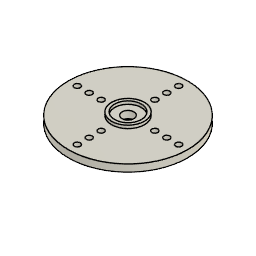
Savöx_SH_0255 MG_micro_servo_horn (Autodesk Fusion 360 design; units mm, degrees)
description: Spur Gear; Module: 0.217; Num Teeth: 21; Pressure Angle: 20.0; Backlash: 0.00 mm
part number: 2026-07-12-11-53-48-100
Autodesk Fusion 360 part; units mm, degrees
sketch "Horn body" plane through (0, 0, 0) normal (0, 0, 1) x (1, 0, 0)
  circle A0 centre (0, 0) radius 10
  dimension "d1" = 20
  constraint coincident A0.centre origin
  measures "d1" diameter of A0
extrude "Extrude1" add sketch "Horn body" along normal blind 1.2 makes body 1
sketch "Connector" plane through (0, 0, 0) normal (0, 0, -1) x (1, 0, 0)
  circle A0 centre (0, 0) radius 10
  circle A1 centre (0, 0) radius 3.5
  dimension "d5" = 7
  constraint coincident A0.centre A1.centre
  measures "d5" diameter of A1
extrude "Extrude2" add sketch "Connector" along normal blind 3 contours A1 bodies 1
sketch "Screw hole" plane through (0, 0, 1.2) normal (0, 0, 1) x (-1, 0, 0)
  circle A0 centre (0, 0) radius 10
  circle A1 centre (0, 0) radius 2.75
  circle A2 centre (0, 0) radius 2.25
  circle A3 centre (0, 0) radius 1
  dimension "d8" = 5.5
  dimension "d9" = 4.5
  dimension "d10" = 2
  constraint coincident A0.centre A1.centre
  constraint concentric A2 A3
  measures "d8" diameter of A1
  measures "d9" diameter of A2
  measures "d10" diameter of A3
extrude "Extrude3" add sketch "Screw hole" along normal blind 0.5 contours A1 bodies 1
extrude "Extrude4" cut sketch "Screw hole" against normal blind 1.2 contours A3 bodies 1
sketch "Top small holes" plane through (0, 0, 1.2) normal (0, 0, 1) x (-1, 0, 0)
  circle A0 centre (0, 0) radius 10
  circle A1 centre (0, 0) radius 2.75
  circle A2 centre (0, -8.5) radius 0.5
  circle A3 centre (0, -6.5) radius 0.5
  circle A4 centre (0, -4.5) radius 0.5
  dimension "d15" = 1
  dimension "d16" = 1
  dimension "d17" = 1
  dimension "d19" = 8.5
  dimension "d20" = 6.5
  dimension "d21" = 4.5
  measures "d15" diameter of A2
  measures "d16" diameter of A3
  measures "d17" diameter of A4
  measures "d19" distance of A0.centre A2.centre
  measures "d20" distance of A0.centre A3.centre
  measures "d21" distance of A0.centre A4.centre
extrude "Extrude5" cut sketch "Top small holes" against normal blind 1.2 contours A2 | A3 | A4 bodies 1
pattern_circular "C-Pattern1" count 4 over 360 about axis through (0, 0, 1.75) along (0, 0, 1) of "Extrude5"
sketch "Base Circle" plane through (0, 0, 0) normal (0, 0, 1) x (1, 0, 0) in component "Savöx SH 0255 MG Micro Servo Gear"
  circle A0 centre (0, 0) radius 2.0274
extrude "Extrude1'" add sketch "Base Circle" along normal blind 3 separate body makes body 2 in component "Savöx SH 0255 MG Micro Servo Gear"
sketch "Gear Tooth" plane through (0, 0, 0) normal (0, 0, 1) x (1, 0, 0) in component "Savöx SH 0255 MG Micro Servo Gear"
  spline S0 degree 5 poles (2.1325, -0.1918) (2.1335, -0.1919) (2.1355, -0.1921) (2.1386, -0.1922) (2.1427, -0.1923) (2.1478, -0.1921) (2.1529, -0.1919) (2.1581, -0.1915) (2.1632, -0.191) (2.1683, -0.1906) (2.1735, -0.1901) (2.1787, -0.1895) (2.1838, -0.1889) (2.189, -0.1882) (2.1941, -0.1875) (2.1993, -0.1867) (2.2045, -0.1858) (2.2097, -0.1849) (2.2148, -0.1839) (2.22, -0.1829) (2.2252, -0.1818) (2.2304, -0.1807) (2.2356, -0.1796) (2.2407, -0.1784) (2.2459, -0.1772) (2.2511, -0.1759) (2.2563, -0.1746) (2.2615, -0.1732) (2.2667, -0.1718) (2.2719, -0.1703) (2.2771, -0.1689) (2.2823, -0.1674) (2.2875, -0.1658) (2.2927, -0.1642) (2.2979, -0.1626) (2.3031, -0.1609) (2.3083, -0.1592) (2.3134, -0.1575) (2.3186, -0.1557) (2.3238, -0.1539) (2.329, -0.152) (2.3342, -0.1502) (2.3394, -0.1482) (2.3446, -0.1463) (2.3498, -0.1443) (2.355, -0.1423) (2.3602, -0.1403) (2.3654, -0.1382) (2.3705, -0.1361) (2.3757, -0.1339) (2.3809, -0.1317) (2.3861, -0.1295) (2.3913, -0.1273) (2.3964, -0.125) (2.4016, -0.1227) (2.4068, -0.1204) (2.412, -0.118) (2.4171, -0.1156) (2.4223, -0.1132) (2.4275, -0.1107) (2.4326, -0.1082) (2.4378, -0.1057) (2.4429, -0.1032) (2.4481, -0.1006) (2.4532, -0.098) (2.4584, -0.0953) (2.4635, -0.0927) (2.4687, -0.09) (2.4738, -0.0872) (2.479, -0.0845) (2.4841, -0.0817) (2.4882, -0.0794) (2.4913, -0.0777) (2.4933, -0.0766) (2.4943, -0.076) knots 0 0 0 0 0 0 0.01428571 0.02857143 0.04285714 0.05714286 0.07142857 0.08571429 0.1 0.11428571 0.12857143 0.14285714 0.15714286 0.17142857 0.18571429 0.2 0.21428571 0.22857143 0.24285714 0.25714286 0.27142857 0.28571429 0.3 0.31428571 0.32857143 0.34285714 0.35714286 0.37142857 0.38571429 0.4 0.41428571 0.42857143 0.44285714 0.45714286 0.47142857 0.48571429 0.5 0.51428571 0.52857143 0.54285714 0.55714286 0.57142857 0.58571429 0.6 0.61428571 0.62857143 0.64285714 0.65714286 0.67142857 0.68571429 0.7 0.71428571 0.72857143 0.74285714 0.75714286 0.77142857 0.78571429 0.8 0.81428571 0.82857143 0.84285714 0.85714286 0.87142857 0.88571429 0.9 0.91428571 0.92857143 0.94285714 0.95714286 0.97142857 0.98571429 1 1 1 1 1 1
  spline S1 degree 5 poles (2.1325, 0.1918) (2.1335, 0.1919) (2.1355, 0.1921) (2.1386, 0.1922) (2.1427, 0.1923) (2.1478, 0.1921) (2.1529, 0.1919) (2.1581, 0.1915) (2.1632, 0.191) (2.1683, 0.1906) (2.1735, 0.1901) (2.1787, 0.1895) (2.1838, 0.1889) (2.189, 0.1882) (2.1941, 0.1875) (2.1993, 0.1867) (2.2045, 0.1858) (2.2097, 0.1849) (2.2148, 0.1839) (2.22, 0.1829) (2.2252, 0.1818) (2.2304, 0.1807) (2.2356, 0.1796) (2.2407, 0.1784) (2.2459, 0.1772) (2.2511, 0.1759) (2.2563, 0.1746) (2.2615, 0.1732) (2.2667, 0.1718) (2.2719, 0.1703) (2.2771, 0.1689) (2.2823, 0.1674) (2.2875, 0.1658) (2.2927, 0.1642) (2.2979, 0.1626) (2.3031, 0.1609) (2.3083, 0.1592) (2.3134, 0.1575) (2.3186, 0.1557) (2.3238, 0.1539) (2.329, 0.152) (2.3342, 0.1502) (2.3394, 0.1482) (2.3446, 0.1463) (2.3498, 0.1443) (2.355, 0.1423) (2.3602, 0.1403) (2.3654, 0.1382) (2.3705, 0.1361) (2.3757, 0.1339) (2.3809, 0.1317) (2.3861, 0.1295) (2.3913, 0.1273) (2.3964, 0.125) (2.4016, 0.1227) (2.4068, 0.1204) (2.412, 0.118) (2.4171, 0.1156) (2.4223, 0.1132) (2.4275, 0.1107) (2.4326, 0.1082) (2.4378, 0.1057) (2.4429, 0.1032) (2.4481, 0.1006) (2.4532, 0.098) (2.4584, 0.0953) (2.4635, 0.0927) (2.4687, 0.09) (2.4738, 0.0872) (2.479, 0.0845) (2.4841, 0.0817) (2.4882, 0.0794) (2.4913, 0.0777) (2.4933, 0.0766) (2.4943, 0.076) knots 0 0 0 0 0 0 0.01428571 0.02857143 0.04285714 0.05714286 0.07142857 0.08571429 0.1 0.11428571 0.12857143 0.14285714 0.15714286 0.17142857 0.18571429 0.2 0.21428571 0.22857143 0.24285714 0.25714286 0.27142857 0.28571429 0.3 0.31428571 0.32857143 0.34285714 0.35714286 0.37142857 0.38571429 0.4 0.41428571 0.42857143 0.44285714 0.45714286 0.47142857 0.48571429 0.5 0.51428571 0.52857143 0.54285714 0.55714286 0.57142857 0.58571429 0.6 0.61428571 0.62857143 0.64285714 0.65714286 0.67142857 0.68571429 0.7 0.71428571 0.72857143 0.74285714 0.75714286 0.77142857 0.78571429 0.8 0.81428571 0.82857143 0.84285714 0.85714286 0.87142857 0.88571429 0.9 0.91428571 0.92857143 0.94285714 0.95714286 0.97142857 0.98571429 1 1 1 1 1 1
  arc A0 (2.4943, -0.076) -> (2.4943, 0.076) centre (0, 0) ccw
  line L0 (2.0093, -0.1807) -> (2.1325, -0.1918)
  line L1 (2.0093, 0.1807) -> (2.1325, 0.1918)
  line L2 (2.0093, -0.1807) -> (2.0093, 0.1807)
  point P0 (2.1579, -0.1915)
  point P1 (2.1836, -0.1889)
  point P2 (2.2093, -0.1849)
  point P3 (2.2351, -0.1797)
  point P4 (2.261, -0.1733)
  point P5 (2.287, -0.1659)
  point P6 (2.3129, -0.1576)
  point P7 (2.3389, -0.1484)
  point P8 (2.3649, -0.1384)
  point P9 (2.3908, -0.1275)
  point P10 (2.4168, -0.1158)
  point P11 (2.4427, -0.1033)
  point P12 (2.4685, -0.09)
  point P13 (2.1579, 0.1915)
  point P14 (2.1836, 0.1889)
  point P15 (2.2093, 0.1849)
  point P16 (2.2351, 0.1797)
  point P17 (2.261, 0.1733)
  point P18 (2.287, 0.1659)
  point P19 (2.3129, 0.1576)
  point P20 (2.3389, 0.1484)
  point P21 (2.3649, 0.1384)
  point P22 (2.3908, 0.1275)
  point P23 (2.4168, 0.1158)
  point P24 (2.4427, 0.1033)
  point P25 (2.4685, 0.09)
extrude "Extrude2'" add sketch "Gear Tooth" along normal blind 3 bodies 2 in component "Savöx SH 0255 MG Micro Servo Gear"
fillet "Fillet1" radius 0.1 2 edges at (2.0193, -0.1816, 1.5) (2.0193, 0.1816, 1.5) on bodies 2 in component "Savöx SH 0255 MG Micro Servo Gear"
pattern_circular "C-Pattern1'" count 21 over 360 about axis through (0, 0, 0) along (0, 0, 1) of "Extrude2'", "Fillet1" in component "Savöx SH 0255 MG Micro Servo Gear"
sketch "Diametrial Pitch Circle" plane through (0, 0, 0) normal (0, 0, 1) x (1, 0, 0) in component "Savöx SH 0255 MG Micro Servo Gear"
  circle A0 centre (0, 0) radius 2.2785 construction
move_body "Move1" bodies 2 to x (1, 0, 0) y (0, 1, 0) z (0, 0, 1) at (0, 0, -3) in component "Savöx SH 0255 MG Micro Servo Gear"
combine "Combine1" operation cut target body 1 tool bodies 2 keep tools
component "Savöx SH 0255 MG Micro Servo Gear" placed x (1, 0, 0) y (0, 1, 0) z (0, 0, 1) at (0, 0, 0)
named bodies: "Savöx SH 0255 MG Micro Servo Horn", "Savöx SH 0255 MG Micro Servo Gear"
